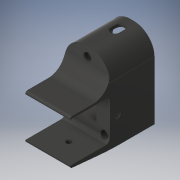
# Autodesk Inventor part: linear_actuator_holder
Saved by Autodesk Inventor 2019.4 (Build 234330000, 330)
## iProperties
Created: 2020-09-27
Part Number: linear_actuator_holder
Material: Generic
Document SubType Name: Modeling
Designer: deanv
Density: 1 g/cm^3
Appearance: Smooth - Black
Author: deanv
Autodesk Inventor part; units mm, degrees
note: some values were not read from the file. Chosen so that the rebuilt part matches the saved one: direction of "Hole1"; edges of "Fillet6".
ref_plane "YZ Plane" through (0, 0, 0) normal (1, 0, 0) x (0, 1, 0)
ref_plane "XZ Plane" through (0, 0, 0) normal (0, 1, 0) x (-1, 0, 0)
ref_plane "XY Plane" through (0, 0, 0) normal (0, 0, 1) x (1, 0, 0)
sketch "Sketch1" plane through (0, 0, 0) normal (0, 0, 1) x (1, 0, 0)
  line L0 (20, -37.4) -> (-20, -37.4) construction
  line L1 (-20, -37.4) -> (-20, 37.4) construction
  line L2 (-20, 37.4) -> (20, 37.4) construction
  line L3 (20, 37.4) -> (20, -37.4) construction
  line L4 (20, -37.4) -> (-20, 37.4) construction
  line L5 (-20, -37.4) -> (20, 37.4) construction
  line L6 (0, 37.4) -> (0, -37.4) construction
  line L7 (8.75, -22.4) -> (-8.75, -22.4)
  line L8 (-8.75, -22.4) -> (-8.75, -4.9)
  line L9 (-8.75, -4.9) -> (8.75, -4.9)
  line L10 (8.75, -4.9) -> (8.75, -22.4)
  line L11 (8.75, -22.4) -> (-8.75, -4.9) construction
  line L12 (-8.75, -22.4) -> (8.75, -4.9) construction
  line L13 (-20, 37.4) -> (20, 37.4)
  line L14 (20, 37.4) -> (20, -37.4)
  line L15 (20, -37.4) -> (-20, -37.4)
  line L16 (-20, -37.4) -> (-20, 37.4)
  line L17 (22.5, -39.9) -> (-22.5, -39.9)
  line L18 (-22.5, -39.9) -> (-22.5, 39.9)
  line L19 (-22.5, 39.9) -> (22.5, 39.9)
  line L20 (22.5, 39.9) -> (22.5, -39.9)
  line L21 (22.5, -39.9) -> (-22.5, 39.9) construction
  line L22 (-22.5, -39.9) -> (22.5, 39.9) construction
  line L23 (-22.5, -39.9) -> (22.5, -39.9) construction
  line L24 (22.5, -39.9) -> (22.5, 5.1) construction
  line L25 (22.5, 5.1) -> (-22.5, 5.1) construction
  line L26 (-22.5, 5.1) -> (-22.5, -39.9) construction
  line L27 (-22.5, 8.85) -> (22.5, 8.85) construction
  line L28 (22.5, 8.85) -> (22.5, -36.15) construction
  line L29 (22.5, -36.15) -> (-22.5, -36.15) construction
  line L30 (-22.5, -36.15) -> (-22.5, 8.85) construction
  line L31 (-22.5, 8.85) -> (22.5, -36.15) construction
  line L32 (22.5, 8.85) -> (-22.5, -36.15) construction
  line L33 (22.5, -36.15) -> (-22.5, -36.15)
  line L34 (-22.5, -36.15) -> (-22.5, -33.65)
  line L35 (-22.5, -33.65) -> (22.5, -33.65)
  line L36 (22.5, -33.65) -> (22.5, -36.15)
  line L37 (22.5, 8.85) -> (-22.5, 8.85)
  line L38 (-22.5, 8.85) -> (-22.5, 6.35)
  line L39 (-22.5, 6.35) -> (22.5, 6.35)
  line L40 (22.5, 6.35) -> (22.5, 8.85)
  point P0 (0, 0)
  point P1 (-17, -28.974)
  point P2 (17, -28.974)
  point P3 (0, 30.4)
  point P4 (0, -13.65)
  dimension "d0" = 40
  dimension "d1" = 74.8
  dimension "d2" = 34
  dimension "d3" = 17
  dimension "d4" = 8.426
  dimension "d5" = 8.426
  dimension "d6" = 17.5
  dimension "d7" = 17.5
  dimension "d8" = 15
  dimension "d9" = 45
  dimension "d10" = 79.8
  dimension "d11" = 45
  dimension "d12" = 7
  dimension "d24" = 45
  dimension "d25" = 2.5
  dimension "d26" = 2.5
  constraints: 82 end point, 16 parallel, 10 midpoint, 8 horizontal, 8 perpendicular, 6 point on line
  measures "d0" distance of L1.end L2.end
  measures "d1" distance of L0.end L1.end
  measures "d2" distance of point (17, -28.974) point (-17, -28.974)
  measures "d3" distance from line of L6 point (-17, -28.974)
  measures "d4" distance from line of L0 point (17, -28.974)
  measures "d5" distance from line of L0 point (-17, -28.974)
  measures "d6" distance of L8.end L9.end
  measures "d7" distance of L7.end L8.end
  measures "d8" distance between parallel lines of L0 L7
  measures "d9" distance of L18.end L19.end
  measures "d10" distance of L19.end L17.start
  measures "d11" distance of L24.end L23.end
  measures "d12" distance from line of L2 point (0, 30.4)
  measures "d24" distance of L27.end L28.end
  measures "d25" distance of L33.end L34.end
  measures "d26" distance of L38.end L37.end
sketch "Sketch1 outline for Extrusion1" plane through (0, 0, 0) normal (0, 0, 1) x (1, 0, 0)
  line L0 (-20, -37.4) -> (20, -37.4)
  line L1 (-20, 37.4) -> (-20, -37.4)
  line L2 (20, -37.4) -> (20, 37.4)
  line L3 (20, 37.4) -> (-20, 37.4)
  line L4 (8.75, -4.9) -> (8.75, -22.4)
  line L5 (-8.75, -4.9) -> (8.75, -4.9)
  line L6 (-8.75, -22.4) -> (-8.75, -4.9)
  line L7 (8.75, -22.4) -> (-8.75, -22.4)
extrude "Extrusion1" add sketch "Sketch1 outline for Extrusion1" against normal blind 20
sketch "Sketch1 outline for Extrusion2" plane through (0, 0, 0) normal (0, 0, 1) x (1, 0, 0)
  line L0 (22.5, -39.9) -> (-22.5, -39.9)
  line L1 (22.5, 39.9) -> (22.5, -39.9)
  line L2 (-22.5, -39.9) -> (-22.5, 39.9)
  line L3 (-22.5, 39.9) -> (22.5, 39.9)
  line L4 (-20, -37.4) -> (20, -37.4)
  line L5 (20, -37.4) -> (20, 37.4)
  line L6 (20, 37.4) -> (-20, 37.4)
  line L7 (-20, 37.4) -> (-20, -37.4)
extrude "Extrusion2" add sketch "Sketch1 outline for Extrusion2" against normal blind 45
hole "Hole1" at (-17, -28.974, 0) at (17, -28.974, 0) at (0, 30.4, 0) direction (0, 0, -1) diameter 4.134 depth 20 counterbore diameter 7.5 counterbore depth 4 thread size "M5x0.8" class "6H" standard "ISO Metric profile"
sketch "Sketch1 outline for Extrusion3" plane through (0, 0, 0) normal (0, 0, 1) x (1, 0, 0)
  line L0 (22.5, -36.15) -> (-22.5, -36.15)
  line L1 (-22.5, -36.15) -> (-22.5, -33.65)
  line L2 (-22.5, -33.65) -> (22.5, -33.65)
  line L3 (22.5, -33.65) -> (22.5, -36.15)
  line L4 (22.5, 6.35) -> (22.5, 8.85)
  line L5 (-22.5, 6.35) -> (22.5, 6.35)
  line L6 (-22.5, 8.85) -> (-22.5, 6.35)
  line L7 (22.5, 8.85) -> (-22.5, 8.85)
extrude "Extrusion3" add sketch "Sketch1 outline for Extrusion3" along normal blind 40
fillet "Fillet1" radius 6 2 edges at (-20, -37.4, -32.5) (20, -37.4, -32.5)
fillet "Fillet2" radius 21 2 edges at (-20, 37.4, -32.5) (20, 37.4, -32.5)
fillet "Fillet3" radius 21 2 edges at (-22.5, 39.9, -22.5) (22.5, 39.9, -22.5)
fillet "Fillet4" radius 17 1 edges at (0, 8.85, 0)
loft "Loft1" add section 1 edges at (0, -36.15, 0) (-22.5, -38.025, 0) (0, -39.9, 0) (22.5, -38.025, 0) section 2 edges at (0, -36.15, 40) (22.5, -34.9, 40) (0, -33.65, 40) (-22.5, -34.9, 40)
fillet "Fillet5" radius 250 1 edges at (0, -39.9, 0)
fillet "Fillet6" radius 2 2 edges at (0, 8.85, 40) (0, -36.15, 40)
sketch "Sketch2" plane through (-22.5, -33.65, 0) normal (0, 1, 0) x (1, 0, 0)
  line L0 (45, -40) -> (0, -40) construction
  line L1 (0, 0) -> (45, 0) construction
  line L2 (45, 0) -> (45, -40) construction
  line L3 (45, -40) -> (0, -40) construction
  line L4 (0, -40) -> (0, 0) construction
  line L5 (3.5, -40) -> (43.5, -40) construction
  line L6 (43.5, -40) -> (43.5, 0) construction
  line L7 (43.5, 0) -> (3.5, 0) construction
  line L8 (3.5, 0) -> (3.5, -40) construction
  line L9 (3.5, 0) -> (43.5, -40) construction
  line L10 (3.5, -40) -> (43.5, 0) construction
  point P0 (22.5, 0)
  point P1 (23.5, -20)
  dimension "d39" = 40
  dimension "d40" = 3.5
  constraints: 20 end point, 4 parallel, 2 horizontal, 2 perpendicular, 2 point on line, 1 midpoint
  measures "d39" distance between parallel lines of L6 L8
  measures "d40" distance between parallel lines of L4 L8
hole "Hole2" at (1, -33.65, 20) direction (0, -1, 0) diameter 5 end through all
sketch "Sketch3" plane through (-8.75, -22.4, 0) normal (1, 0, 0) x (0, 0, -1)
  line L0 (0, 17.5) -> (20, 17.5) projected
  line L1 (0, 0) -> (8, 0) construction
  line L2 (8, 0) -> (8, 17.5) construction
  line L3 (8, 17.5) -> (0, 17.5) construction
  line L4 (0, 17.5) -> (0, 0) construction
  line L5 (8, 0) -> (0, 0) construction
  line L6 (0, 0) -> (0, 9) construction
  line L7 (0, 9) -> (8, 9) construction
  line L8 (8, 9) -> (8, 0) construction
  point P0 (0, 22.4)
  dimension "d48" = 8
  dimension "d49" = 9
  constraints: 16 end point, 4 parallel, 2 horizontal, 2 perpendicular, 2 point on line, 1 coincident
  measures "d48" distance of L3.end L2.end
  measures "d49" distance of L5.end L6.end
hole "Hole3" at (-8.75, -13.4, -8) direction (-1, 0, 0) diameter 6.5 end through all both
fillet "Fillet7" radius 4 2 edges at (0, 6.35, 0) (0, -33.65, 0)
sketch "Sketch4" plane through (-1.5, 39.9, 0) normal (0, 1, 0) x (1, 0, 0)
  line L0 (3, 45) -> (3, 0) projected
  line L1 (0, 45) -> (3, 45) construction
  line L2 (3, 45) -> (3, 20) construction
  line L3 (3, 20) -> (0, 20) construction
  line L4 (0, 20) -> (0, 45) construction
  line L5 (0, 20) -> (3, 20) construction
  line L6 (3, 20) -> (3, 29.981) construction
  line L7 (3, 29.981) -> (0, 29.981)
  line L8 (0, 29.981) -> (0, 20) construction
  line L9 (1.5, 32.481) -> (1.5, 27.481)
  line L10 (-3, 32.481) -> (-3, 27.481)
  line L11 (6, 27.481) -> (6, 32.481)
  arc A0 (6, 32.481) -> (-3, 32.481) centre (1.5, 32.481) ccw
  arc A1 (-3, 27.481) -> (6, 27.481) centre (1.5, 27.481) ccw
  point P0 (1.5, 0)
  point P1 (1.5, 29.981)
  dimension "d58" = 25
  dimension "d59" = 9.981
  dimension "d60" = 2.5
  dimension "d61" = 9
  constraints: 24 end point, 5 parallel, 4 point on circle, 4 tangent, 3 perpendicular, 2 centre point, 2 horizontal, 2 midpoint, 2 point on line
  measures "d58" distance of L1.end L2.end
  measures "d59" distance of L6.end L5.end
  measures "d60" distance of point (1.5, 29.981) L9.end
  measures "d61" diameter of A1
sketch "Sketch4 outline for Extrusion4" plane through (-1.5, 39.9, 0) normal (0, 1, 0) x (1, 0, 0)
  arc A0 (6, 32.481) -> (-3, 32.481) centre (1.5, 32.481) ccw
  line L0 (6, 27.481) -> (6, 32.481)
  arc A1 (-3, 27.481) -> (6, 27.481) centre (1.5, 27.481) ccw
  line L1 (-3, 32.481) -> (-3, 27.481)
extrude "Extrusion4" cut sketch "Sketch4 outline for Extrusion4" against normal blind 40
equation "\"d3\" = 0.5 * d2"
equation "\"d5\" = d4"
equation "\"d6\" = d7"
body "Solid1"
